Autodesk Fusion 360 part; units mm, degrees
(part 2 of 2)
sketch "Sketch7" plane through (0, 0, 0) normal (0, 0, -1) x (1, 0, 0)
  circle A0 centre (44.6077, 77.2628) radius 2.35
  circle A1 centre (-44.6077, -77.2628) radius 2.35
  circle A2 centre (89.2154, 0) radius 2.35
  circle A3 centre (-44.6077, 77.2628) radius 2.35
  circle A4 centre (-89.2154, 0) radius 2.35
  circle A5 centre (44.6077, -77.2628) radius 2.35
  line L0 (34, 37.5) -> (34, -37.5)
  line L1 (24, -37.5) -> (24, 37.5)
  circle A6 centre (109.2154, 0) radius 7
  circle A7 centre (-109.2154, 0) radius 7
  circle A8 centre (54.6077, 94.5833) radius 7
  circle A9 centre (54.6077, -94.5833) radius 7
  circle A10 centre (-54.6077, -94.5833) radius 7
  circle A11 centre (-54.6077, 94.5833) radius 7
  line L2 (54.6077, 109.3333) -> (-54.6077, 109.3333)
  arc A12 (-54.6077, 109.3333) -> (-67.3816, 101.9583) centre (-54.6077, 94.5833) ccw
  line L3 (-67.3816, 101.9583) -> (-121.9893, 7.375)
  arc A13 (-121.9893, 7.375) -> (-121.9893, -7.375) centre (-109.2154, 0) ccw
  line L4 (-121.9893, -7.375) -> (-67.3816, -101.9583)
  arc A14 (-67.3816, -101.9583) -> (-54.6077, -109.3333) centre (-54.6077, -94.5833) ccw
  line L5 (-54.6077, -109.3333) -> (54.6077, -109.3333)
  arc A15 (54.6077, -109.3333) -> (67.3816, -101.9583) centre (54.6077, -94.5833) ccw
  line L6 (67.3816, -101.9583) -> (121.9893, -7.375)
  arc A16 (121.9893, -7.375) -> (121.9893, 7.375) centre (109.2154, 0) ccw
  line L7 (121.9893, 7.375) -> (67.3816, 101.9583)
  arc A17 (67.3816, 101.9583) -> (54.6077, 109.3333) centre (54.6077, 94.5833) ccw
  circle A18 centre (-71.8801, 41.5) radius 2.25
  circle A19 centre (71.8801, 41.5) radius 2.25
  circle A20 centre (0, -83) radius 2.25
  circle A21 centre (-71.8801, 41.5) radius 2.25
  arc A22 (34, 37.5) -> (24, 37.5) centre (29, 37.5) ccw
  arc A23 (24, -37.5) -> (34, -37.5) centre (29, -37.5) ccw
  circle A24 centre (73.4654, 5) radius 2.85
  circle A25 centre (-32.4026, -66.1229) radius 2.85
  circle A26 centre (-73.4654, -5) radius 2.85
  circle A27 centre (-41.0628, 61.1229) radius 2.85
  circle A28 centre (32.4026, -66.1229) radius 2.85
  circle A29 centre (41.0628, 61.1229) radius 2.85
  circle A30 centre (73.4654, -5) radius 2.85
  circle A31 centre (-41.0628, -61.1229) radius 2.85
  circle A32 centre (-73.4654, 5) radius 2.85
  circle A33 centre (-32.4026, 66.1229) radius 2.85
  circle A34 centre (41.0628, -61.1229) radius 2.85
  circle A35 centre (32.4026, 66.1229) radius 2.85
  circle A36 centre (-0.25, 75.9996) radius 2.85
  dimension "d127" = 4.5
  dimension "d128" = 4.5
  dimension "d129" = 4.5
  dimension "d156" = 83
  dimension "d157" = 83
  dimension "d158" = 83
  constraint concentric A18 A21
  measures "d127" diameter of A18
  measures "d128" diameter of A19
  measures "d129" diameter of A20
  measures "d156" distance of A20.centre origin
  measures "d157" distance of A18.centre origin
  measures "d158" distance of A19.centre origin
extrude "Extrude19" cut sketch "Sketch7" against normal blind 4 contours A18 A21 | A19 | A20 bodies 1
copy_body "Body->Comp1" bodies 3 removing the originals makes body 4 in component "foot"
sketch "Sketch8" plane through (0, 0, 0) normal (0, 0, -1) x (1, 0, 0)
  circle A0 centre (-71.8801, 41.5) radius 2.25
  circle A1 centre (71.8801, 41.5) radius 2.25
  circle A2 centre (0, -83) radius 2.25
  circle A3 centre (44.6077, 77.2628) radius 2.35
  circle A4 centre (-44.6077, -77.2628) radius 2.35
  circle A5 centre (89.2154, 0) radius 2.35
  circle A6 centre (-44.6077, 77.2628) radius 2.35
  circle A7 centre (-89.2154, 0) radius 2.35
  circle A8 centre (44.6077, -77.2628) radius 2.35
  line L0 (24, -37.5) -> (24, 37.5)
  arc A9 (34, 37.5) -> (24, 37.5) centre (29, 37.5) ccw
  line L1 (34, 37.5) -> (34, -37.5)
  arc A10 (24, -37.5) -> (34, -37.5) centre (29, -37.5) ccw
  circle A11 centre (-0.25, 75.9996) radius 2.85
  circle A12 centre (73.4654, 5) radius 2.85
  circle A13 centre (-32.4026, -66.1229) radius 2.85
  circle A14 centre (-73.4654, -5) radius 2.85
  circle A15 centre (-41.0628, 61.1229) radius 2.85
  circle A16 centre (32.4026, -66.1229) radius 2.85
  circle A17 centre (41.0628, 61.1229) radius 2.85
  circle A18 centre (73.4654, -5) radius 2.85
  circle A19 centre (-41.0628, -61.1229) radius 2.85
  circle A20 centre (-73.4654, 5) radius 2.85
  circle A21 centre (-32.4026, 66.1229) radius 2.85
  circle A22 centre (41.0628, -61.1229) radius 2.85
  circle A23 centre (32.4026, 66.1229) radius 2.85
  circle A24 centre (109.2154, 0) radius 7
  circle A25 centre (-109.2154, 0) radius 7
  circle A26 centre (54.6077, 94.5833) radius 7
  circle A27 centre (54.6077, -94.5833) radius 7
  circle A28 centre (-54.6077, -94.5833) radius 7
  circle A29 centre (-54.6077, 94.5833) radius 7
  line L2 (54.6077, 109.3333) -> (-54.6077, 109.3333)
  arc A30 (-54.6077, 109.3333) -> (-67.3816, 101.9583) centre (-54.6077, 94.5833) ccw
  line L3 (-67.3816, 101.9583) -> (-121.9893, 7.375)
  arc A31 (-121.9893, 7.375) -> (-121.9893, -7.375) centre (-109.2154, 0) ccw
  line L4 (-121.9893, -7.375) -> (-67.3816, -101.9583)
  arc A32 (-67.3816, -101.9583) -> (-54.6077, -109.3333) centre (-54.6077, -94.5833) ccw
  line L5 (-54.6077, -109.3333) -> (54.6077, -109.3333)
  arc A33 (54.6077, -109.3333) -> (67.3816, -101.9583) centre (54.6077, -94.5833) ccw
  line L6 (67.3816, -101.9583) -> (121.9893, -7.375)
  arc A34 (121.9893, -7.375) -> (121.9893, 7.375) centre (109.2154, 0) ccw
  line L7 (121.9893, 7.375) -> (67.3816, 101.9583)
  arc A35 (67.3816, 101.9583) -> (54.6077, 109.3333) centre (54.6077, 94.5833) ccw
  line L8 (-81.8549, 5.4043) -> (-88.2154, 9.0765)
  line L9 (-90.2154, 9.0765) -> (-96.5759, 5.4043)
  line L10 (-97.5759, 3.6722) -> (-97.5759, -3.6722)
  line L11 (-96.5759, -5.4043) -> (-90.2154, -9.0765)
  line L12 (-88.2154, -9.0765) -> (-81.8549, -5.4043)
  line L13 (-80.8549, -3.6722) -> (-80.8549, 3.6722)
  circle A36 centre (-89.2154, 0) radius 3.85
  arc A37 (-88.2154, 9.0765) -> (-90.2154, 9.0765) centre (-89.2154, 7.3445) ccw
  arc A38 (-80.8549, 3.6722) -> (-81.8549, 5.4043) centre (-82.8549, 3.6722) ccw
  arc A39 (-81.8549, -5.4043) -> (-80.8549, -3.6722) centre (-82.8549, -3.6722) ccw
  arc A40 (-90.2154, -9.0765) -> (-88.2154, -9.0765) centre (-89.2154, -7.3445) ccw
  arc A41 (-97.5759, -3.6722) -> (-96.5759, -5.4043) centre (-95.5759, -3.6722) ccw
  arc A42 (-96.5759, 5.4043) -> (-97.5759, 3.6722) centre (-95.5759, 3.6722) ccw
  point P0 (-89.2154, 0)
  dimension "d178" = 8.3605
  dimension "d179" = 7.7
  dimension "d180" = 2
  constraint coincident P0 A7.centre
  constraint tangent L9 A37
  constraint tangent L8 A37
  constraint tangent L8 A38
  constraint tangent L13 A38
  constraint equal A37 A38
  constraint tangent L12 A39
  constraint tangent L13 A39
  constraint equal A37 A39
  constraint tangent L11 A40
  constraint tangent L12 A40
  constraint equal A37 A40
  constraint tangent L10 A41
  constraint tangent L11 A41
  constraint equal A37 A41
  constraint tangent L9 A42
  constraint tangent L10 A42
  constraint equal A37 A42
  measures "d178" distance of P0 L13
  measures "d179" diameter of A36
  measures "d180" radius of A37
extrude "Extrude24" cut sketch "Sketch8" against normal blind 0.6 contours L8 L9 L10 L11 L12 L13 A37 A38 A39 A40 A41 A42 bodies 1
pattern_circular "C-Pattern1" count 6 over 360 about axis through (0, 0, 1.75) along (0, 0, 1) of "Extrude24"
component "foot" placed x (1, 0, 0) y (0, 1, 0) z (0, 0, 1) at (0, 0, 0)
hidden bodies 4
equation "d1 = base_diameter / 2"
equation "base_diameter = 260 mm"
equation "d3 = base_height"
equation "base_height = 6.5 mm"
equation "d19 = -base_height"
equation "d21 = -base_height"
equation "d25 = base_height / 2"
equation "d37 = -base_height"
equation "internal_height = 90 mm"
equation "d54 = internal_height"
equation "d56 = internal_height"
equation "d82 = -base_height"
equation "d149 = -base_height"
equation "d152 = -base_height"
equation "d178 = ( ( 16.321 / 2 ) * 1 ) * 1 mm + 0.2 mm"
named bodies: "Base", "foot", "Battery Stop"

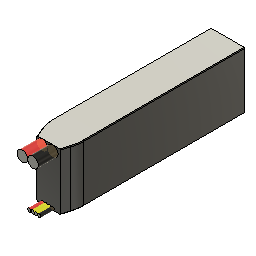
design "battery"
Autodesk Fusion 360 part; units mm, degrees
sketch "Sketch1" plane through (0, 0, 0) normal (0, 0, 1) x (1, 0, 0)
  line L0 (0, 0) -> (26, 0)
  line L1 (26, 0) -> (26, 137)
  line L2 (26, 137) -> (0, 137)
  line L3 (0, 137) -> (0, 0)
  dimension "d1" = 26
  dimension "d2" = 137
  constraint horizontal L0
  constraint vertical L1
  constraint horizontal L2
  constraint vertical L3
  constraint coincident L0.start L3.end
  measures "d1" distance of L0.start L0.end
  measures "d2" distance of L0.start L2.end
extrude "Extrude1" add sketch "Sketch1" along normal blind 43 makes body 1
sketch "Sketch2" plane through (0, 0, 0) normal (0, -1, 0) x (1, 0, 0)
  line L0 (0, 0) -> (26, 0)
  line L1 (26, 0) -> (26, 43)
  line L2 (26, 43) -> (0, 43)
  line L3 (0, 43) -> (0, 0)
  line L4 (21, 35) -> (5, 35) construction
  line L5 (5, 35) -> (5, 51) construction
  line L6 (5, 51) -> (21, 51) construction
  line L7 (21, 51) -> (21, 35) construction
  line L8 (21, 35) -> (5, 51) construction
  line L9 (5, 35) -> (21, 51) construction
  line L10 (13, 43) -> (5, 35) construction
  line L11 (13, 43) -> (21, 35) construction
  circle A0 centre (9, 39) radius 4
  circle A1 centre (17, 39) radius 4
  point P0 (13, 43)
  dimension "d5" = 16
  dimension "d6" = 16
  constraint horizontal L4
  constraint perpendicular L4 L5
  constraint parallel L4 L6
  constraint parallel L5 L7
  constraint coincident L8 P0
  constraint coincident L9 P0
  constraint midpoint L2 P0
  constraint coincident P0 L10.start
  constraint midpoint L10 A0.centre
  constraint tangent L2 A0
  constraint midpoint L11 A1.centre
  constraint tangent L2 A1
  measures "d5" distance of L5.end L6.end
  measures "d6" distance of L4.end L5.end
extrude "Extrude2" add sketch "Sketch2" along normal blind 15 separate body contours A0 | A1 makes body 2
sketch "Sketch3" plane through (0, 0, 0) normal (0, -1, 0) x (1, 0, 0)
  line L0 (0, 0) -> (26, 0)
  line L1 (26, 0) -> (26, 43)
  line L2 (26, 43) -> (0, 43)
  line L3 (0, 43) -> (0, 0)
  line L4 (18, 2.5) -> (8, 2.5) construction
  line L5 (8, 2.5) -> (8, -2.5) construction
  line L6 (8, -2.5) -> (18, -2.5) construction
  line L7 (18, -2.5) -> (18, 2.5) construction
  line L8 (18, 2.5) -> (8, -2.5) construction
  line L9 (8, 2.5) -> (18, -2.5) construction
  line L10 (8, 2.5) -> (8, 0)
  line L11 (8, 1.25) -> (9.25, 1.25) construction
  circle A0 centre (9.25, 1.25) radius 1.25
  circle A1 centre (11.75, 1.25) radius 1.25
  circle A2 centre (14.25, 1.25) radius 1.25
  circle A3 centre (16.75, 1.25) radius 1.25
  point P0 (13, 0)
  dimension "d9" = 10
  dimension "d10" = 5
  dimension "d11" = 1.25
  constraint horizontal L4
  constraint perpendicular L4 L5
  constraint parallel L4 L6
  constraint parallel L5 L7
  constraint coincident L8 P0
  constraint coincident L9 P0
  constraint midpoint L0 P0
  constraint midpoint L5 L10.end
  constraint midpoint L10 L11.start
  constraint perpendicular L5 L11
  constraint coincident L11.end A0.centre
  constraint tangent L4 A0
  measures "d9" distance of L5.end L6.end
  measures "d10" distance of L4.end L5.end
  measures "d11" distance of L11.start L11.end
extrude "Extrude3" add sketch "Sketch3" along normal blind 10 separate body contours A0 | A1 | A2 | A3 makes body 3
chamfer "Chamfer1" distance 3 distance2 10 1 edges at (26, 0, 21.5) measured on face at (8.6667, 0, 14.3333) on bodies 1
chamfer "Chamfer2" distance 12 distance2 5 1 edges at (0, 0, 21.5) measured on face at (0, 91.3333, 14.3333) on bodies 1
fillet "Fillet1" radius 30 2 edges at (0, 12, 21.5) (26, 10, 21.5) on bodies 1
chamfer "Chamfer3" distance 0.5 distance2 0.5 12 edges at (25.682, 10.0467, 0) (26, 75.7015, 0) (23.8674, 2.8913, 0) (0, 77.5, 0) (0.5826, 12.1165, 0) (3.6538, 3.2308, 0) (0.5826, 12.1165, 43) (0, 77.5, 43) (3.6538, 3.2308, 43) (26, 75.7015, 43) (23.8674, 2.8913, 43) (25.682, 10.0467, 43) 1 faces at (17.3333, 137, 14.3333) measured on face at (25.9843, 13.4317, 14.3333) measured on face at (26, 55.2687, 14.3333) measured on face at (23.5783, 1.9275, 14.3333) measured on face at (0, 97.3333, 14.3333) measured on face at (1.8284, 7.687, 28.6667) measured on face at (3.2051, 4.3077, 28.6667) measured on face at (1.8284, 7.687, 28.6667) measured on face at (17.3333, 56.4677, 43) measured on face at (3.2051, 4.3077, 28.6667) measured on face at (17.3333, 56.4677, 43) measured on face at (23.5783, 1.9275, 14.3333) measured on face at (25.9843, 13.4317, 14.3333) on bodies 1

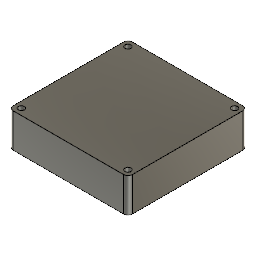
design "noctua_fan_80mm"
Autodesk Fusion 360 part; units mm, degrees
box "BoxPrimitive1" add length 80 width 80 height 23 placed x (0, -1, 0) y (1, 0, 0) z (0, 0, 1) at (0, 0, 0)
fillet "Fillet1" radius 3 4 edges at (0, -80, 11.5) (80, -80, 11.5) (80, 0, 11.5) (0, 0, 11.5)
sketch "Sketch2" plane through (0, 0, 23) normal (0, 0, 1) x (-1, 0, 0)
  arc A0 (-3, 0) -> (0, 3) centre (-3, 3) ccw
  line L0 (0, 3) -> (0, 77)
  arc A1 (0, 77) -> (-3, 80) centre (-3, 77) ccw
  line L1 (-3, 80) -> (-77, 80)
  arc A2 (-77, 80) -> (-80, 77) centre (-77, 77) ccw
  line L2 (-80, 77) -> (-80, 3)
  arc A3 (-80, 3) -> (-77, 0) centre (-77, 3) ccw
  line L3 (-77, 0) -> (-3, 0)
  circle A4 centre (-75.75, 75.75) radius 2
  circle A5 centre (-75.75, 4.25) radius 2
  circle A6 centre (-4.25, 75.75) radius 2
  circle A7 centre (-4.25, 4.25) radius 2
  dimension "d8" = 4
  dimension "d9" = 4
  dimension "d10" = 4
  dimension "d11" = 4
  dimension "d12" = 4.25
  dimension "d13" = 4.25
  dimension "d14" = 4.25
  dimension "d15" = 4.25
  dimension "d16" = 4.25
  dimension "d17" = 4.25
  dimension "d18" = 4.25
  dimension "d19" = 4.25
  measures "d8" diameter of A4
  measures "d9" diameter of A5
  measures "d10" diameter of A6
  measures "d11" diameter of A7
  measures "d12" distance of L1 A4.centre
  measures "d13" distance of L2 A4.centre
  measures "d14" distance of L3 A5.centre
  measures "d15" distance of L2 A5.centre
  measures "d16" distance of L3 A7.centre
  measures "d17" distance of L0 A7.centre
  measures "d18" distance of L1 A6.centre
  measures "d19" distance of L0 A6.centre
extrude "Extrude1" cut sketch "Sketch2" against normal blind 35 contours A4 | A5 | A6 | A7
